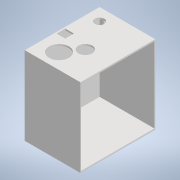
# Autodesk Inventor part: Outer Casing
Saved by Autodesk Inventor 2021 (Build 250183000, 183)
## iProperties
Created: 2022-05-16
Part Number: Outer Casing
Material: Generic
Document SubType Name: Modeling
Designer: techv
Density: 1 g/cm^3
Appearance: Default
Author: techv
Autodesk Inventor part; units mm, degrees
ref_plane "YZ Plane" through (0, 0, 0) normal (1, 0, 0) x (0, 1, 0)
ref_plane "XZ Plane" through (0, 0, 0) normal (0, 1, 0) x (-1, 0, 0)
ref_plane "XY Plane" through (0, 0, 0) normal (0, 0, 1) x (1, 0, 0)
sketch "Sketch1" plane through (0, 0, 0) normal (0, 1, 0) x (-1, 0, 0)
  line L0 (-225, 302.5) -> (225, 302.5)
  line L1 (225, 302.5) -> (225, -302.5)
  line L2 (225, -302.5) -> (-225, -302.5)
  line L3 (-225, -302.5) -> (-225, 302.5)
  line L4 (-225, 302.5) -> (225, -302.5) construction
  line L5 (225, 302.5) -> (-225, -302.5) construction
  line L6 (-219, 296.5) -> (219, 296.5)
  line L7 (219, 296.5) -> (219, -296.5)
  line L8 (219, -296.5) -> (-219, -296.5)
  line L9 (-219, -296.5) -> (-219, 296.5)
  line L10 (-219, 296.5) -> (219, -296.5) construction
  line L11 (219, 296.5) -> (-219, -296.5) construction
  line L12 (-219, 296.5) -> (-225, 296.5)
  line L13 (-219, 296.5) -> (-213, 296.5) construction
  line L14 (-219, -296.5) -> (-225, -296.5)
  line L15 (-219, -296.5) -> (-213, -296.5) construction
  point P0 (0, 0)
  dimension "d0" = 450
  dimension "d1" = 605
  dimension "d2" = 438
  dimension "d3" = 593
  dimension "d4" = 6
  dimension "d5" = 180
  dimension "d6" = 6
  dimension "d7" = 180
  constraints: 32 end point, 5 horizontal, 4 midpoint, 4 parallel, 3 perpendicular, 2 collinear
  measures "d0" distance of L1.end L2.end
  measures "d1" distance of L0.end L1.end
  measures "d2" distance of L7.end L8.end
  measures "d3" distance of L6.end L7.end
  measures "d4" distance of L6.start L12.end
  measures "d5" angle of L12 L13
  measures "d6" distance of L8.end L14.end
  measures "d7" angle of L14 L15
extrude "Extrusion1" add sketch "Sketch1" along normal blind 635 contours L0 L1 L2 L3 L14 L8 L7 L6 L12
sketch "Sketch2" plane through (-219, 0, -296.5) normal (0, 0, 1) x (1, 0, 0)
  line L0 (0, 635) -> (444, 635) projected
  line L1 (444, 0) -> (444, 635) projected
  line L2 (0, 635) -> (444, 635)
  line L3 (444, 635) -> (444, 623)
  line L4 (444, 623) -> (0, 623)
  line L5 (0, 623) -> (0, 635)
  line L6 (0, 0) -> (444, 0)
  line L7 (444, 0) -> (444, 12)
  line L8 (444, 12) -> (0, 12)
  line L9 (0, 12) -> (0, 0)
  point P0 (219, 0)
  dimension "d10" = 12
  dimension "d13" = 12
  constraints: 16 end point, 4 parallel, 2 horizontal, 2 perpendicular, 2 point on line
  measures "d10" distance of L2.end L3.end
  measures "d13" distance of L7.end L6.end
extrude "Extrusion2" add sketch "Sketch2" along normal up to surface (593 mm away)
sketch "Sketch3" plane through (0, 635, 0) normal (0, 1, 0) x (1, 0, 0)
  circle A0 centre (-73, -177.5) radius 80
  line L0 (-225, 302.5) -> (-225, -302.5) projected
  line L1 (-225, -302.5) -> (225, -302.5) projected
  circle A1 centre (-125, 202.5) radius 37.5
  line L2 (225, 302.5) -> (-225, 302.5) projected
  line L3 (-213, -57.5) -> (-143, -57.5)
  line L4 (-143, -57.5) -> (-143, 12.5)
  line L5 (-143, 12.5) -> (-213, 12.5)
  line L6 (-213, 12.5) -> (-213, -57.5)
  line L7 (-213, -57.5) -> (-143, 12.5) construction
  line L8 (-143, -57.5) -> (-213, 12.5) construction
  circle A2 centre (15, -52.5) radius 55
  line L9 (225, -302.5) -> (225, 302.5) projected
  line L10 (-53, 85.5) -> (-213, 85.5)
  line L11 (-213, 85.5) -> (-213, 290.5)
  line L12 (-213, 290.5) -> (-53, 290.5)
  line L13 (-53, 290.5) -> (-53, 85.5)
  line L14 (-53, 85.5) -> (-213, 290.5) construction
  line L15 (-213, 85.5) -> (-53, 290.5) construction
  point P0 (0, 0)
  point P1 (-178, -22.5)
  point P2 (-133, 188)
  dimension "d14" = 160
  dimension "d15" = 152
  dimension "d16" = 125
  dimension "d17" = 75
  dimension "d18" = 100
  dimension "d19" = 100
  dimension "d20" = 325
  dimension "d21" = 47
  dimension "d22" = 70
  dimension "d23" = 70
  dimension "d24" = 110
  dimension "d25" = 210
  dimension "d26" = 250
  dimension "d37" = 205
  dimension "d38" = 160
  dimension "d39" = 12
  dimension "d40" = 12
  constraints: 24 end point, 4 midpoint, 4 parallel, 3 centre point, 2 horizontal, 2 perpendicular
  measures "d14" diameter of A0
  measures "d15" distance from line of L0 A0.centre
  measures "d16" distance from line of L1 A0.centre
  measures "d17" diameter of A1
  measures "d18" distance from line of L2 A1.centre
  measures "d19" distance from line of L0 A1.centre
  measures "d20" distance from line of L2 point (-178, -22.5)
  measures "d21" distance from line of L0 point (-178, -22.5)
  measures "d22" distance of L3.end L4.end
  measures "d23" distance of L4.end L5.end
  measures "d24" diameter of A2
  measures "d25" distance from line of L9 A2.centre
  measures "d26" distance from line of L1 A2.centre
  measures "d37" distance of L12.end L10.start
  measures "d38" distance of L11.end L12.end
  measures "d39" distance between parallel lines of L0 L11
  measures "d40" distance between parallel lines of L2 L12
extrude "Extrusion3" cut sketch "Sketch3" against normal blind 100 contours A0 | A1 | L6 L5 L4 L3 | A2 | L10 L11 L12 L13
sketch "Sketch4" plane through (225, 0, -302.5) normal (0, 0, -1) x (-1, 0, 0)
  line L0 (255, 587.5) -> (410, 587.5)
  line L1 (410, 587.5) -> (410, 502.5)
  line L2 (410, 502.5) -> (255, 502.5)
  line L3 (255, 502.5) -> (255, 587.5)
  line L4 (255, 587.5) -> (410, 502.5) construction
  line L5 (410, 587.5) -> (255, 502.5) construction
  line L6 (450, 0) -> (450, 635) projected
  line L7 (0, 635) -> (450, 635) projected
  point P0 (225, 0)
  point P1 (332.5, 545)
  dimension "d31" = 155
  dimension "d32" = 85
  dimension "d33" = 40
  dimension "d34" = 90
  constraints: 12 end point, 2 midpoint, 2 parallel, 1 horizontal, 1 perpendicular
  measures "d31" distance of L1.end L2.end
  measures "d32" distance of L0.end L1.end
  measures "d33" distance between parallel lines of L6 L1
  measures "d34" distance from line of point (332.5, 545) L7
extrude "Extrusion4" cut sketch "Sketch4" against normal blind 100
sketch "Sketch5" plane through (-219, 12, 296.5) normal (1, 0, 0) x (0, 0, -1)
  line L0 (22.5, 561) -> (332.5, 561)
  line L1 (332.5, 561) -> (332.5, 529)
  line L2 (332.5, 529) -> (22.5, 529)
  line L3 (22.5, 529) -> (22.5, 561)
  line L4 (22.5, 561) -> (332.5, 529) construction
  line L5 (332.5, 561) -> (22.5, 529) construction
  line L6 (0, 0) -> (0, 611) projected
  line L7 (593, 611) -> (0, 611) projected
  point P0 (296.5, -12)
  point P1 (177.5, 545)
  dimension "d41" = 22.5
  dimension "d42" = 310
  dimension "d43" = 32
  dimension "d44" = 82
  constraints: 12 end point, 2 midpoint, 2 parallel, 1 horizontal, 1 perpendicular
  measures "d41" distance between parallel lines of L6 L3
  measures "d42" distance of L1.end L2.end
  measures "d43" distance of L0.end L1.end
  measures "d44" distance between parallel lines of L7 L2
extrude "Extrusion5" add sketch "Sketch5" along normal blind 260
sketch "Sketch6" plane through (-219, 12, 296.5) normal (1, 0, 0) x (0, 0, -1)
  line L0 (423, 458) -> (593, 458)
  line L1 (593, 458) -> (593, 446)
  line L2 (593, 446) -> (423, 446)
  line L3 (423, 446) -> (423, 458)
  line L4 (423, 458) -> (593, 446) construction
  line L5 (593, 458) -> (423, 446) construction
  line L6 (593, 611) -> (0, 611) projected
  line L7 (593, 0) -> (593, 611) projected
  point P0 (296.5, -12)
  point P1 (508, 452)
  dimension "d47" = 170
  dimension "d48" = 12
  dimension "d49" = 165
  dimension "d50" = 0
  constraints: 12 end point, 2 midpoint, 2 parallel, 1 horizontal, 1 perpendicular
  measures "d47" distance of L1.end L2.end
  measures "d48" distance of L2.end L0.start
  measures "d49" distance between parallel lines of L6 L2
  measures "d50" distance between parallel lines of L7 L1
extrude "Extrusion6" add sketch "Sketch6" along normal blind 220
sketch "Sketch7" plane through (-219, 12, -296.5) normal (0, 1, 0) x (1, 0, 0)
  circle A0 centre (119, -353) radius 50
  line L0 (444, 0) -> (444, -593) projected
  line L1 (444, -593) -> (0, -593) projected
  point P0 (219, -296.5)
  dimension "d53" = 100
  dimension "d54" = 325
  dimension "d55" = 240
  constraints: 1 centre point
  measures "d53" diameter of A0
  measures "d54" distance from line of L0 A0.centre
  measures "d55" distance from line of L1 A0.centre
extrude "Extrusion7" add sketch "Sketch7" along normal blind 10
body "Solid1"
